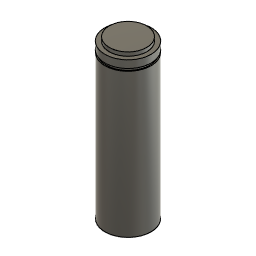
18650 v2 (Autodesk Fusion 360 design; units mm, degrees)
Autodesk Fusion 360 part; units mm, degrees
sketch "Sketch4" plane through (0, 0, 0) normal (0, 0, 1) x (1, 0, 0)
cylinder "CylinderPrimitive1" add diameter 18.4 height 20 placed x (1, 0, 0) y (0, 0, -1) z (0, 1, 0) at (-6, 0, 15) makes body 1
move_face "MoveFace1" by (0, -38, 0) 1 faces at (-6.9682, 0, 8.1968) on bodies 1
sketch "Sketch6" plane through (0, 0, 0) normal (0, 0, 1) x (1, 0, 0)
sketch "Sketch7" plane through (0, 20, 0) normal (0, 1, 0) x (-1, 0, 0)
  circle A0 centre (6, 15) radius 9.2
  circle A1 centre (6, 15) radius 8.75
  dimension "d7" = 17.5
  constraint concentric A0 A1
  measures "d7" diameter of A1
extrude "Extrude1" add sketch "Sketch7" along normal blind 1 contours A1 bodies 1
sketch "Sketch8" plane through (0, 21, 0) normal (0, 1, 0) x (-1, 0, 0)
  circle A0 centre (6, 15) radius 8.75
  circle A1 centre (6, 15) radius 9.25
  dimension "d10" = 18.5
  constraint concentric A0 A1
  measures "d10" diameter of A1
extrude "Extrude2" add sketch "Sketch8" along normal blind 3 contours A0 | A1 bodies 1
sketch "Sketch9" plane through (0, 0, 0) normal (1, 0, 0) x (0, 0, -1)
sketch "Sketch10" plane through (0, 0, 0) normal (0, 0, 1) x (1, 0, 0)
sketch "Sketch11" plane through (0, 24, 0) normal (0, 1, 0) x (-1, 0, 0)
  circle A0 centre (6, 15) radius 9.25
  circle A1 centre (6, 15) radius 7.5
  dimension "d13" = 15
  constraint concentric A0 A1
  measures "d13" diameter of A1
extrude "Extrude3" add sketch "Sketch11" along normal blind 1.5 contours A1 bodies 1
sketch "Sketch12" plane through (0, -38, 0) normal (0, -1, 0) x (1, 0, 0)
  circle A0 centre (-6, 15) radius 9.2
  circle A1 centre (-6, 15) radius 8.5
  constraint concentric A0 A1
extrude "Extrude4" cut sketch "Sketch12" against normal blind 0.5 contours A1 bodies 1
fillet "Fillet1" radius 9.2 1 edges at (-13.9248, -38, 18.0737) on bodies 1
fillet "Fillet2" radius 0.25 1 edges at (-14.5774, -38, 11.6731) on bodies 1
copy_body "Body->Comp1" bodies 1 removing the originals makes body 2 in component "18650"
component "18650" placed x (1, 0, 0) y (0, 1, 0) z (0, 0, 1) at (0, 0, 0)
